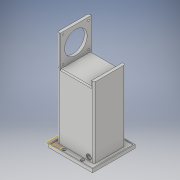
# Autodesk Inventor part: suport motor
Saved by Autodesk Inventor 2019 (Build 230136000, 136)
## iProperties
Created: 2018-08-16
Part Number: suport motor
Material: Genérico
Document SubType Name: Modeling
Designer: Albert Garangou Culebras
Density: 1 g/cm^3
Appearance: Valor por defecto
Author: Albert Garangou Culebras
Autodesk Inventor part; units mm, degrees
ref_plane "YZ Plane" through (0, 0, 0) normal (1, 0, 0) x (0, 1, 0)
ref_plane "XZ Plane" through (0, 0, 0) normal (0, 1, 0) x (-1, 0, 0)
ref_plane "XY Plane" through (0, 0, 0) normal (0, 0, 1) x (1, 0, 0)
sketch "Boceto1" plane through (0, 0, 0) normal (0, 1, 0) x (-1, 0, 0)
  line L0 (0, 0) -> (0, -55)
  line L1 (0, -55) -> (-65, -55)
  line L2 (-65, -55) -> (-65, 0)
  line L3 (-65, 0) -> (0, 0)
  dimension "d0" = 55
  dimension "d1" = 65
  constraints: 8 end point, 3 perpendicular, 1 vertical
  measures "d0" distance of L0.start L0.end
  measures "d1" distance of L0.end L1.end
extrude "Extrusión1" add sketch "Boceto1" along normal blind 120
sketch "Boceto2" plane through (0, 120, 0) normal (0, 1, 0) x (1, 0, 0)
  line L0 (0, 55) -> (0, 0) projected
  line L1 (65, 0) -> (65, 55) projected
  line L2 (65, 0) -> (65, 55)
  line L3 (0, 55) -> (5, 55)
  line L4 (5, 0) -> (5, 55)
  line L5 (60, 0) -> (60, 55)
  line L6 (5, 55) -> (5, 0)
  line L7 (0, 55) -> (5, 55)
  line L8 (0, 0) -> (5, 0)
  line L9 (60, 55) -> (65, 55)
  line L10 (60, 0) -> (65, 0)
  dimension "d4" = 65
  dimension "d5" = 55
  constraints: 18 end point, 1 parallel, 1 perpendicular
  measures "d4" distance of L0.end L1.start
  measures "d5" distance of L1.start L1.end
extrude "Extrusión2" add sketch "Boceto2" along normal blind 55 contours L3 L4 L8 L0
sketch "Boceto3" plane through (0, 120, 0) normal (0, 1, 0) x (1, 0, 0)
  line L0 (0, 55) -> (65, 55) projected
  line L1 (65, 0) -> (60, 0)
  line L2 (60, 0) -> (60, 55)
  line L3 (60, 55) -> (65, 55)
  line L4 (65, 55) -> (65, 0)
  point P0 (0, 0)
  constraints: 8 end point, 2 parallel, 1 horizontal, 1 perpendicular, 1 point on line
extrude "Extrusión3" add sketch "Boceto3" along normal blind 10
sketch "Boceto4" plane through (0, 0, -55) normal (-1, 0, 0) x (0, 0, 1)
  line L0 (0, 120) -> (55, 120) projected
  line L1 (0, 120) -> (55, 120)
  line L2 (0, 175) -> (55, 175)
  line L3 (55, 175) -> (55, 120)
  line L4 (55, 120) -> (0, 120)
  line L5 (0, 120) -> (0, 175)
  circle A0 centre (27.5, 147.5) radius 20
  line L6 (0, 120) -> (0, 175) projected
  line L7 (55, 175) -> (0, 175) projected
  line L8 (0, 175) -> (55, 175) projected
  line L9 (0, 0) -> (0, 175) projected
  line L10 (0, 175) -> (5, 175)
  line L11 (0, 175) -> (0, 170)
  circle A1 centre (5, 170) radius 1.6
  line L12 (55, 0) -> (55, 175) projected
  line L13 (55, 170) -> (55, 168)
  circle A2 centre (50, 170) radius 1.6
  circle A3 centre (50, 125) radius 1.6
  circle A4 centre (5, 125) radius 1.6
  dimension "d11" = 40
  dimension "d22" = 5
  dimension "d23" = 5
  dimension "d24" = 3.2
  dimension "d29" = 3.2
  dimension "d36" = 3.2
  dimension "d37" = 3.2
  constraints: 16 end point, 5 centre point, 4 point on line, 3 equal length, 1 horizontal, 1 perpendicular
  measures "d11" diameter of A0
  measures "d22" distance of L2.start L10.end
  measures "d23" distance of L2.start L11.end
  measures "d24" diameter of A1
  measures "d29" diameter of A4
  measures "d36" diameter of A2
  measures "d37" diameter of A3
extrude "Extrusión4" cut sketch "Boceto4" against normal blind 10 contours A0 | A1 | A2 | A3 | A4
sketch "Boceto6" plane through (0, 0, -55) normal (-1, 0, 0) x (0, 0, 1)
  circle A0 centre (50, 125) radius 1.6 projected
  circle A1 centre (50, 125) radius 3
  circle A2 centre (50, 170) radius 3
  circle A3 centre (5, 170) radius 3
  circle A4 centre (5, 125) radius 1.6 projected
  circle A5 centre (5, 125) radius 3
  point P0 (55, 0)
  dimension "d38" = 6
  dimension "d39" = 6
  dimension "d40" = 6
  dimension "d41" = 6
  constraints: 4 centre point, 2 coincident
  measures "d38" diameter of A1
  measures "d39" diameter of A2
  measures "d40" diameter of A3
  measures "d41" diameter of A5
extrude "Extrusión5" cut sketch "Boceto6" against normal blind 2.75
sketch "Boceto7" plane through (0, 0, 0) normal (0, -1, 0) x (1, 0, 0)
  line L0 (0, -55) -> (65, -55)
  line L1 (65, -55) -> (65, 0)
  line L2 (65, 0) -> (0, 0)
  line L3 (0, 0) -> (0, -55)
  line L4 (65, 10) -> (70, 10)
  line L5 (0, -65) -> (-5, -65)
  line L6 (-5, -65) -> (72, -65)
  line L7 (72, -65) -> (72, 10)
  line L8 (72, 10) -> (-5, 10)
  line L9 (-5, 10) -> (-5, -65)
  line L10 (0, -55) -> (65, -55) projected
  line L11 (32.5, -55) -> (65, -55)
  line L12 (0, -55) -> (32.5, -55)
  circle A0 centre (16.25, -59.25) radius 1.5
  circle A1 centre (48.75, -59.25) radius 1.5
  circle A2 centre (16.25, 4.25) radius 1.5
  circle A3 centre (48.75, 4.25) radius 1.5
  dimension "d49" = 5
  dimension "d50" = 10
  dimension "d51" = 5
  dimension "d65" = 3
  dimension "d66" = 3
  dimension "d69" = 3
  constraints: 24 end point, 4 centre point, 4 parallel, 2 collinear, 2 horizontal, 2 perpendicular, 1 midpoint
  measures "d49" distance of L4.start L4.end
  measures "d50" distance of L0.start L5.start
  measures "d51" distance of L5.start L5.end
  measures "d65" diameter of A0
  measures "d66" diameter of A1
  measures "d69" diameter of A3
ref_plane "Plano de trabajo2" through (0, 5, 0) normal (0, 1, 0) x (1, 0, 0)
sketch "Boceto8" plane through (0, 5, 0) normal (0, 1, 0) x (1, 0, 0)
  line L0 (-5, 65) -> (72, 65) projected
  line L1 (-5, 65) -> (-5, 63.5)
  line L2 (-5, -10) -> (-5, 65) projected
  line L3 (-5, 63.5) -> (-3.5, 63.5)
  line L4 (72, -10) -> (70.5, -10)
  line L5 (72, -10) -> (-5, -10) projected
  line L6 (70.5, -10) -> (70.5, -8.5)
  line L7 (70.5, -8.5) -> (-3.5, -8.5)
  line L8 (-3.5, -8.5) -> (-3.5, 63.5)
  line L9 (-3.5, 63.5) -> (70.5, 63.5)
  line L10 (70.5, 63.5) -> (70.5, -8.5)
  line L11 (72, 65) -> (-5, 65)
  line L12 (-5, 65) -> (-5, -10)
  line L13 (-5, -10) -> (72, -10)
  line L14 (72, -10) -> (72, 65)
  point P0 (0, 0)
  dimension "d58" = 1.5
  dimension "d59" = 1.5
  dimension "d60" = 1.5
  dimension "d61" = 1.5
  constraints: 24 end point, 4 parallel, 4 perpendicular, 2 horizontal, 2 point on line
  measures "d58" distance of L0.start L1.end
  measures "d59" distance of L1.end L3.end
  measures "d60" distance of L4.start L4.end
  measures "d61" distance of L4.end L6.end
extrude "Extrusión7" add sketch "Boceto8" along normal blind 1 contours L0 L14 L4 L6 L10 L9 L3 L1 | L3 L8 L7 L6 L5 L2
extrude "Extrusión8" add sketch "Boceto7" against normal blind 5
sketch "Boceto9" plane through (0, 5, 0) normal (0, 1, 0) x (1, 0, 0)
  circle A0 centre (16.25, 59.25) radius 1.5 projected
  circle A1 centre (16.25, 59.25) radius 3
  circle A2 centre (48.75, 59.25) radius 1.5 projected
  circle A3 centre (48.75, 59.25) radius 3
  circle A4 centre (48.75, -4.25) radius 1.5 projected
  circle A5 centre (48.75, -4.25) radius 3
  circle A6 centre (16.25, -4.25) radius 1.5 projected
  circle A7 centre (16.25, -4.25) radius 3
  point P0 (0, 0)
  dimension "d72" = 6
  dimension "d73" = 6
  dimension "d74" = 6
  dimension "d75" = 6
  constraints: 4 centre point, 4 coincident
  measures "d72" diameter of A1
  measures "d73" diameter of A3
  measures "d74" diameter of A5
  measures "d75" diameter of A7
extrude "Extrusión9" cut sketch "Boceto9" against normal blind 3
sketch "Boceto10" plane through (0, 175, -55) normal (-1, 0, 0) x (0, 0, 1)
  line L0 (0, -55) -> (0, -54.5)
  line L1 (0, -170) -> (0, 0) projected
  line L2 (0, -54.5) -> (0, -55.5)
  line L3 (0, -55.5) -> (55, -55.5)
  line L4 (55, -170) -> (55, 0) projected
  line L5 (55, -54.5) -> (0, -54.5)
  line L6 (55, -54.5) -> (55, -55.5)
  line L7 (55, -55) -> (55, 0) projected
  point P0 (55, -175)
  dimension "d78" = 0.5
  dimension "d79" = 1
  constraints: 10 end point, 3 point on line, 1 collinear, 1 perpendicular
  measures "d78" distance of L0.start L0.end
  measures "d79" distance of L0.end L2.end
extrude "Extrusión10" cut sketch "Boceto10" against normal blind 1
sketch "Boceto11" plane through (0, 120, 0) normal (0, 1, 0) x (1, 0, 0)
  line L0 (60, 55) -> (60, 0) projected
  line L1 (60, 27.5) -> (52, 27.5)
  line L2 (52, 27.5) -> (59, 27.5)
  circle A0 centre (55.5, 27.5) radius 3.5
  point P0 (0, 0)
  dimension "d82" = 8
  dimension "d83" = 7
  constraints: 4 end point, 2 midpoint, 1 horizontal, 1 horizontal alignment, 1 point on line, 2 other
  measures "d82" distance of L1.start L1.end
  measures "d83" distance of L1.end L2.end
extrude "Extrusión11" cut sketch "Boceto11" against normal blind 109
sketch "Boceto12" plane through (0, 175, 0) normal (0, 0, 1) x (1, 0, 0)
  line L0 (5, -55) -> (60, -55) projected
  line L1 (60, -55) -> (60, -175)
  line L2 (59, -55) -> (59, -164) projected
  line L3 (52, -55) -> (59, -55) projected
  line L4 (55.5, -55) -> (55.5, -164)
  circle A0 centre (55.5, -164) radius 3.5
  point P0 (0, -175)
  dimension "d86" = 109
  dimension "d87" = 7
  constraints: 4 end point, 1 centre point, 1 coincident, 1 midpoint, 1 parallel, 1 vertical
  measures "d86" distance of L4.start L4.end
  measures "d87" diameter of A0
extrude "Extrusión12" cut sketch "Boceto12" against normal blind 508 contours A0
sketch "Boceto13" plane through (0, 120, 0) normal (0, 1, 0) x (1, 0, 0)
  circle A0 centre (55.5, 27.5) radius 3.5 projected
  line L0 (52, 27.5) -> (59, 27.5)
  circle A1 centre (55.5, 27.5) radius 5
  line L1 (50.5, 27.5) -> (50.5, 22.5)
  line L2 (50.5, 22.5) -> (55.5, 22.5)
  line L3 (50.5, 27.5) -> (50.5, 32.5)
  line L4 (50.5, 32.5) -> (55.5, 32.5)
  point P0 (0, 0)
  dimension "d90" = 10
  constraints: 10 end point, 5 point on circle, 2 perpendicular, 2 vertical, 1 centre point, 1 coincident, 1 horizontal, 1 tangent
  measures "d90" diameter of A1
extrude "Extrusión13" cut sketch "Boceto13" against normal blind 1
sketch "Boceto14" plane through (0, 175, 0) normal (0, 0, 1) x (1, 0, 0)
  arc A0 (59, -164) -> (52, -164) centre (55.5, -164) ccw projected
  line L0 (55.5, -164) -> (55.5, -160.5)
  circle A1 centre (55.5, -164) radius 4.5
  point P0 (0, -175)
  dimension "d93" = 9
  constraints: 2 end point, 1 centre point, 1 coincident, 1 point on circle, 1 vertical
  measures "d93" diameter of A1
extrude "Extrusión14" cut sketch "Boceto14" against normal blind 0.8
sketch "Boceto15" plane through (5, 175, -55) normal (0, 0, -1) x (-1, 0, 0)
  circle A0 centre (-50.5, -164) radius 3.5 projected
  line L0 (-47, -164) -> (-50.5, -164)
  circle A1 centre (-50.5, -164) radius 4.5
  point P0 (5, -175)
  dimension "d96" = 9
  constraints: 2 end point, 1 centre point, 1 coincident, 1 horizontal, 1 horizontal alignment, 1 other
  measures "d96" diameter of A1
extrude "Extrusión15" cut sketch "Boceto15" against normal blind 0.8
fillet "Empalme1" radius 3 4 edges at (65, 67.5, 0) (0, 62.25, 0) (65, 67.5, -55) (0, 62.25, -55)
chamfer "Chaflán1" distance 2 angle 45 2 edges at (32.5, 120, 0) (32.5, 120, -55)
